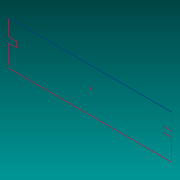
# Autodesk Inventor part: 滑块
Saved by Autodesk Inventor 2021 (Build 250183000, 183)
## iProperties
Created: 2025-04-17
Part Number: 滑块
Material: 常规
Document SubType Name: Modeling
Designer: 86155
Density: 1 g/cm^3
Appearance: 默认
Author: 86155
Autodesk Inventor part; units mm, degrees
ref_plane "YZ Plane" through (0, 0, 0) normal (1, 0, 0) x (0, 1, 0)
ref_plane "XZ Plane" through (0, 0, 0) normal (0, 1, 0) x (-1, 0, 0)
ref_plane "XY Plane" through (0, 0, 0) normal (0, 0, 1) x (1, 0, 0)
ref_plane "工作平面1" through (0, 0, 214.75) normal (0, 0, 1) x (1, 0, 0)
sketch "草图2" plane through (0, 0, 214.75) normal (0, 0, 1) x (1, 0, 0)
  line L0 (15, -0.25) -> (15, -3.75) projected
  line L1 (15, 3.75) -> (15, 0.75) projected
  line L2 (15, 0.75) -> (13.5, 0.75) projected
  line L3 (13.5, 0.75) -> (13.5, -0.25) projected
  line L4 (13.5, -0.25) -> (15, -0.25) projected
  line L5 (27.5, 3.75) -> (-27.5, 3.75) projected
  line L6 (-15, 0.75) -> (-15, 3.75) projected
  line L7 (-15, -3.75) -> (-15, -0.25) projected
  line L8 (-13.5, 0.75) -> (-15, 0.75) projected
  line L9 (-13.5, -0.25) -> (-13.5, 0.75) projected
  line L10 (-15, -0.25) -> (-13.5, -0.25) projected
  line L11 (-15, -4.25) -> (15, -4.25) projected
  line L12 (-15, -3.75) -> (-15, -4.25) projected
  line L13 (15, -4.25) -> (15, -3.75) projected
  line L14 (18, 3.75) -> (18, -8.25)
  line L15 (-18, 3.75) -> (-18, -8.25)
  line L16 (-18, -8.25) -> (18, -8.25)
  point P0 (0, 0)
  dimension "d0" = 12
  dimension "d1" = 3
  dimension "d2" = 12
  dimension "d3" = 3
  constraints: 6 end point, 2 point on line, 1 perpendicular, 1 vertical
  measures "d0" distance of L14.start L14.end
  measures "d1" distance between parallel lines of L1 L14
  measures "d2" distance of L15.start L15.end
  measures "d3" distance between parallel lines of L6 L15
extrude "拉伸1" add sketch "草图2" along normal blind 50 contours L4 L3 L2 L1 L5 L14 L16 L15 L6 L8 L9 L10 L7 L12 L11 L13 L0
sketch "草图3" plane through (-18, -8.25, 214.75) normal (0, -1, 0) x (1, 0, 0)
  line L0 (0, 0) -> (0, 50) projected
  line L1 (0, 0) -> (36, 0) projected
  line L2 (0, 50) -> (14, 50)
  line L3 (14, 50) -> (14, 0)
  line L4 (14, 0) -> (0, 0)
  line L5 (0, 0) -> (0, 50)
  line L6 (0, 50) -> (36, 50) projected
  line L7 (36, 50) -> (22, 50)
  line L8 (22, 50) -> (22, 0)
  line L9 (22, 0) -> (36, 0)
  line L10 (36, 0) -> (36, 50)
  point P0 (18, -214.75)
  dimension "d6" = 14
  dimension "d7" = 14
  constraints: 16 end point, 4 parallel, 2 horizontal, 2 perpendicular, 2 point on line
  measures "d6" distance of L3.end L4.end
  measures "d7" distance of L9.end L8.end
extrude "拉伸2" add sketch "草图3" along normal blind 2 contours L0 L2 L3 L1 | L8 L6 L10 L1
sketch "草图4" plane through (-18, -10.25, 214.75) normal (0, -1, 0) x (1, 0, 0)
  line L0 (0, 50) -> (0, 0) projected
  line L1 (14, 50) -> (0, 50) projected
  line L2 (0, 0) -> (14, 0) projected
  line L3 (36, 50) -> (22, 50) projected
  line L4 (36, 0) -> (36, 50) projected
  line L5 (22, 0) -> (36, 0) projected
  point P0 (18, -214.75)
  point P1 (7, 42)
  point P2 (7, 8)
  point P3 (29, 42)
  point P4 (29, 8)
  dimension "d10" = 7
  dimension "d11" = 8
  dimension "d12" = 8
  dimension "d13" = 7
  dimension "d14" = 8
  dimension "d15" = 7
  dimension "d16" = 7
  dimension "d17" = 8
  measures "d10" distance from line of L0 point (7, 42)
  measures "d11" distance from line of L1 point (7, 42)
  measures "d12" distance from line of L2 point (7, 8)
  measures "d13" distance from line of L0 point (7, 8)
  measures "d14" distance from line of L3 point (29, 42)
  measures "d15" distance from line of L4 point (29, 42)
  measures "d16" distance from line of L4 point (29, 8)
  measures "d17" distance from line of L5 point (29, 8)
hole "孔1" at (-11, -10.25, 256.75) at (-11, -10.25, 222.75) at (11, -10.25, 256.75) at (11, -10.25, 222.75) direction (0, 1, 0) diameter 3.242 depth 3 tip angle 118 thread size "M4x0.7" designation "M4" class "6H" standard "GB Metric profile"
